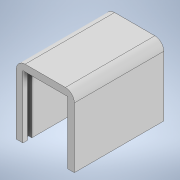
# Autodesk Inventor part: Case_Side
Saved by Autodesk Inventor 2020 (Build 240168000, 168)
## iProperties
Created: 2019-11-07
Part Number: Case_Side
Material: 일반
Document SubType Name: Modeling
Designer: Knowblesse
Density: 1 g/cm^3
Appearance: 기본값
Author: Knowblesse
## iProperties of the stored document _3D 인쇄.ipt
Created: 2019-11-07
Part Number: _3D 인쇄
Material: 일반
Document SubType Name: Modeling
Designer: Knowblesse
Density: 1 g/cm^3
Appearance: 기본값
Author: Knowblesse
Autodesk Inventor part; units mm, degrees
ref_plane "YZ Plane" through (0, 0, 0) normal (1, 0, 0) x (0, 1, 0)
ref_plane "XZ Plane" through (0, 0, 0) normal (0, 1, 0) x (-1, 0, 0)
ref_plane "XY Plane" through (0, 0, 0) normal (0, 0, 1) x (1, 0, 0)
sketch "스케치1" plane through (0, 0, 0) normal (0, 0, 1) x (1, 0, 0)
  line L0 (0, 0) -> (10, 0)
  line L1 (10, 0) -> (10, 12.5)
  line L2 (10, 12.5) -> (0, 12.5)
  line L3 (0, 12.5) -> (0, 0)
  line L4 (-1.5, 14) -> (11.5, 14)
  line L5 (11.5, 14) -> (11.5, -1.5)
  line L6 (11.5, -1.5) -> (-1.5, -1.5)
  line L7 (-1.5, -1.5) -> (-1.5, 14)
  line L8 (0, 0) -> (0, -1.5)
  line L9 (10, 0) -> (10, -1.5)
  line L10 (0, 0) -> (-1.5, 0)
  line L11 (10, 0) -> (11.5, 0)
  dimension "d0" = 10
  dimension "d1" = 12.5
  dimension "d2" = 1.5
  constraints: 24 end point, 6 point on line, 4 parallel, 4 perpendicular, 1 horizontal, 3 other
  measures "d0" distance of L2.end L1.end
  measures "d1" distance of L1.end L0.end
  measures "d2" distance between parallel lines of L2 L4
extrude "돌출1" add sketch "스케치1" along normal blind 20 contours L10 L7 L4 L5 L11 L1 L2 L3 | L8 L6 L7 L10 | L11 L5 L6 L9
sketch "스케치2" plane through (-1.5, -1.5, 0) normal (0, -1, 0) x (1, 0, 0)
  line L0 (0, 0) -> (1.5, 0) projected
  line L1 (1.5, 0) -> (1.5, 20) projected
  line L2 (0, 20) -> (1.5, 20) projected
  line L3 (0, 0) -> (0, 20) projected
  line L4 (1.5, 5.5) -> (0, 5.5)
  line L5 (0, 5.5) -> (0, 6)
  line L6 (0, 6) -> (1.5, 6)
  line L7 (1.5, 6) -> (1.5, 5.5)
  point P0 (1.5, 0)
  point P1 (1.5, 6)
  point P2 (0, 5.5)
  dimension "d5" = 0.5
  dimension "d6" = 5.5
  constraints: 8 end point, 2 parallel, 2 point on line, 1 horizontal, 1 perpendicular
  measures "d5" distance of L4.end L5.end
  measures "d6" distance between parallel lines of L4 L0
extrude "돌출2" cut sketch "스케치2" against normal blind 8 contours L3 L6 L1 L4
fillet "모깎기1" radius 2 2 edges at (-1.5, 14, 10) (11.5, 14, 10)
sketch "스케치3" plane through (10, -1.5, 0) normal (0, -1, 0) x (1, 0, 0)
  line L0 (-10.75, 19) -> (0.75, 19)
  line L1 (0.75, 19) -> (0.75, 18)
  line L2 (0.75, 18) -> (-10.75, 18)
  line L3 (-10.75, 18) -> (-10.75, 19)
  line L4 (-11.5, 6) -> (-10, 6) projected
  line L5 (-10, 6) -> (-10, 20) projected
  line L6 (-11.5, 20) -> (-10, 20) projected
  line L7 (-11.5, 6) -> (-11.5, 20) projected
  line L8 (0, 0) -> (1.5, 0) projected
  line L9 (1.5, 0) -> (1.5, 20) projected
  line L10 (0, 20) -> (1.5, 20) projected
  line L11 (0, 0) -> (0, 20) projected
  point P0 (-10, 0)
  point P1 (-10.75, 20)
  point P2 (-10.75, 18.5)
  point P3 (0.75, 20)
  point P4 (0.75, 18.5)
  dimension "d10" = 1
  dimension "d11" = 1
  constraints: 8 end point, 4 midpoint, 2 parallel, 2 vertical alignment, 1 horizontal, 1 perpendicular
  measures "d10" distance of L2.end L0.start
  measures "d11" distance between parallel lines of L6 L0
extrude "돌출3" cut sketch "스케치3" against normal blind 14.5 contours L0 L5 L2 L3 | L0 L11 L2 L5 | L0 L1 L2 L11
sketch "스케치4" plane through (0, -1.5, 0) normal (1, 0, 0) x (0, 0, -1)
  line L0 (-2.8, 5.5) -> (-1.8, 5.5)
  line L1 (-1.8, 5.5) -> (-1.8, 8.5)
  line L2 (-1.8, 8.5) -> (-2.8, 8.5)
  line L3 (-2.8, 8.5) -> (-2.8, 5.5)
  line L4 (0, 0) -> (-5.5, 0) projected
  line L5 (0, 13.5) -> (0, 0) projected
  point P0 (0, 1.5)
  point P1 (-2.8, 7)
  dimension "d14" = 1
  dimension "d15" = 3
  dimension "d16" = 7
  dimension "d20" = 2.8
  constraints: 8 end point, 2 parallel, 1 horizontal, 1 midpoint, 1 perpendicular
  measures "d14" distance between parallel lines of L3 L1
  measures "d15" distance of L2.end L0.start
  measures "d16" distance from line of L4 point (-2.8, 7)
  measures "d20" distance between parallel lines of L5 L3
extrude "돌출4" add sketch "스케치4" along normal blind 2
